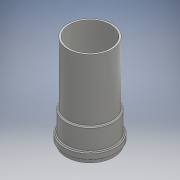
# Autodesk Inventor part: hullPipe
Saved by Autodesk Inventor 2016 (Build 200138000, 138)
## iProperties
Created: 2015-10-11
Part Number: hullPipe
Material: PVC-Piping
Document SubType Name: Modeling
Designer: Artur
Density: 1.4 g/cm^3
Appearance: Smooth - White
Mass: 158.885 g
Surface Area: 1512.99 cm^2
Volume: 149.892 cm^3
Author: Artur
Autodesk Inventor part; units mm, degrees
ref_plane "YZ Plane" through (0, 0, 0) normal (1, 0, 0) x (0, 1, 0)
ref_plane "XZ Plane" through (0, 0, 0) normal (0, 1, 0) x (-1, 0, 0)
ref_plane "XY Plane" through (0, 0, 0) normal (0, 0, 1) x (1, 0, 0)
sketch "Sketch2" plane through (0, 0, 0) normal (1, 0, 0) x (0, 1, 0)
  line L0 (-51.5, 0) -> (-51.5, -160)
  line L1 (-51.5, -160) -> (-55.5, -160)
  line L2 (0, 0) -> (0, -206.7356) construction
  line L3 (-77.4, 0) -> (12.9, 0) construction
  line L4 (-55.5, 0) -> (-55.5, -156)
  line L5 (-55.5, -156) -> (-59.5, -156)
  line L6 (-59.5, -233) -> (-59.5, -224)
  line L7 (-59.5, -224) -> (-64.5, -224)
  line L8 (-64.5, -224) -> (-64.5, -208)
  line L9 (-64.5, -208) -> (-59.5, -208)
  line L10 (-59.5, -208) -> (-59.5, -156)
  line L11 (-55.5, -233) -> (-59.5, -233)
  line L12 (-55.5, -233) -> (-55.5, -220)
  line L13 (-55.5, -220) -> (-60.5, -220)
  line L14 (-60.5, -220) -> (-60.5, -212)
  line L15 (-60.5, -212) -> (-55.5, -212)
  line L16 (-55.5, -212) -> (-55.5, -160)
  line L17 (-55.5, 0) -> (-51.5, 0)
  dimension "d4" = 160
  dimension "d6" = 73
  dimension "d7" = 103
  dimension "d9" = 4
  dimension "d11" = 4
  dimension "d12" = 9
  dimension "d13" = 5
  dimension "d14" = 16
  dimension "d16" = 4
  dimension "d17" = 4
  dimension "d18" = 4
  dimension "d19" = 4
  dimension "d20" = 111
  constraints: 34 end point, 9 perpendicular, 5 vertical, 4 point on line, 1 coincident, 1 collinear, 1 horizontal, 1 parallel
  measures "d4" distance of L0.start L0.end
  measures "d6" distance of L1.end L11.start
  measures "d7" diameter of L0 L2
  measures "d9" distance between parallel lines of L4 L0
  measures "d11" distance between parallel lines of L5 L1
  measures "d12" distance of L6.start L6.end
  measures "d13" distance of L6.end L7.end
  measures "d14" distance of L7.end L8.end
  measures "d16" distance between parallel lines of L9 L15
  measures "d17" distance between parallel lines of L7 L13
  measures "d18" distance between parallel lines of L6 L12
  measures "d19" distance between parallel lines of L14 L8
  measures "d20" diameter of L12 L2
revolve "Revolution1" add sketch "Sketch2" angle 360 about axis through (0, 0, 0) along (0, 0, -1)
fillet "Fillet1" radius 2 2 edges at (0, 55.5, -156) (0, 59.5, -156)
fillet "Fillet2" radius 2 4 edges at (0, 64.5, -208) (0, 59.5, -208) (0, 64.5, -224) (0, 59.5, -224)
equation "\"d11\" = d9"
equation "\"d16\" = d11"
equation "\"d17\" = d11"
equation "\"d18\" = d16"
equation "\"d19\" = d16"
body "Solid2"
